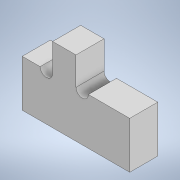
# Autodesk Inventor part: Little Scrap Piece
Saved by Autodesk Inventor 2020 (Build 240168000, 168)
## iProperties
Created: 2020-05-09
Part Number: Little Scrap Piece
Material: Generic
Document SubType Name: Modeling
Designer: Dan Wikman
Density: 1 g/cm^3
Appearance: Default
Autodesk Inventor part; units mm, degrees
ref_plane "YZ Plane" through (0, 0, 0) normal (1, 0, 0) x (0, 1, 0)
ref_plane "XZ Plane" through (0, 0, 0) normal (0, 1, 0) x (-1, 0, 0)
ref_plane "XY Plane" through (0, 0, 0) normal (0, 0, 1) x (1, 0, 0)
sketch "CONTOURS" plane through (0, 0, 0) normal (0, 0, 1) x (1, 0, 0)
  arc A0 (68.6456, 67.1763) -> (76.6456, 67.1763) centre (72.6456, 67.1763) ccw
  line L0 (76.6456, 67.1763) -> (103.1456, 67.1763)
  line L1 (103.1456, 67.1763) -> (103.1456, 37.1763)
  line L2 (103.1456, 37.1763) -> (34.1456, 37.1763)
  line L3 (34.1456, 37.1763) -> (34.1456, 67.1763)
  line L4 (34.1456, 67.1763) -> (45.6456, 67.1763)
  arc A1 (45.6456, 67.1763) -> (53.6456, 67.1763) centre (49.6456, 67.1763) ccw
  line L5 (53.6456, 67.1763) -> (53.6456, 85.1763)
  line L6 (53.6456, 85.1763) -> (68.6456, 85.1763)
  line L7 (68.6456, 85.1763) -> (68.6456, 67.1763)
  constraints: 16 end point, 4 point on circle, 2 centre point
extrude "Extrusion4" add sketch "CONTOURS" along normal blind 18
body "Solid2"
